Autodesk Inventor part; units mm, degrees
(part 2 of 11)
  arc A198 (21.2642, 29.6462) -> (21.4078, 29.7898) centre (21.336, 29.718) ccw
  line L98 (18.542, 32.512) -> (18.542, 37.846)
  arc A199 (18.6436, 37.846) -> (18.4404, 37.846) centre (18.542, 37.846) ccw
  arc A200 (18.4404, 32.512) -> (18.6436, 32.512) centre (18.542, 32.512) ccw
  line L99 (18.542, 37.846) -> (-1.016, 37.846)
  arc A201 (-1.016, 37.9476) -> (-1.016, 37.7444) centre (-1.016, 37.846) ccw
  arc A202 (18.542, 37.7444) -> (18.542, 37.9476) centre (18.542, 37.846) ccw
  line L100 (-1.016, 37.846) -> (-1.016, -0.762)
  arc A203 (-1.1176, -0.762) -> (-0.9144, -0.762) centre (-1.016, -0.762) ccw
  arc A204 (-0.9144, 37.846) -> (-1.1176, 37.846) centre (-1.016, 37.846) ccw
  line L101 (26.162, 10.668) -> (27.432, 10.668)
  arc A205 (27.432, 10.6045) -> (27.432, 10.7315) centre (27.432, 10.668) ccw
  arc A206 (26.162, 10.7315) -> (26.162, 10.6045) centre (26.162, 10.668) ccw
  line L102 (26.162, 26.162) -> (26.162, 27.432)
  arc A207 (26.2255, 27.432) -> (26.0985, 27.432) centre (26.162, 27.432) ccw
  arc A208 (26.0985, 26.162) -> (26.2255, 26.162) centre (26.162, 26.162) ccw
  line L103 (10.668, 26.162) -> (9.398, 26.162)
  arc A209 (9.398, 26.2255) -> (9.398, 26.0985) centre (9.398, 26.162) ccw
  arc A210 (10.668, 26.0985) -> (10.668, 26.2255) centre (10.668, 26.162) ccw
  line L104 (10.668, 10.668) -> (10.668, 9.398)
  arc A211 (10.6045, 9.398) -> (10.7315, 9.398) centre (10.668, 9.398) ccw
  arc A212 (10.7315, 10.668) -> (10.6045, 10.668) centre (10.668, 10.668) ccw
  line L105 (10.668, 26.162) -> (10.922, 26.162)
  arc A213 (10.922, 26.0985) -> (10.922, 26.2255) centre (10.922, 26.162) ccw
  arc A214 (10.668, 26.2255) -> (10.668, 26.0985) centre (10.668, 26.162) ccw
  line L106 (12.954, 26.67) -> (11.176, 26.67)
  arc A215 (11.176, 26.7335) -> (11.176, 26.6065) centre (11.176, 26.67) ccw
  arc A216 (12.954, 26.6065) -> (12.954, 26.7335) centre (12.954, 26.67) ccw
  line L107 (11.176, 26.67) -> (10.668, 26.162)
  arc A217 (10.6231, 26.2069) -> (10.7129, 26.1171) centre (10.668, 26.162) ccw
  arc A218 (11.2209, 26.6251) -> (11.1311, 26.7149) centre (11.176, 26.67) ccw
  line L108 (5.588, 34.036) -> (5.588, 30.48)
  arc A219 (5.5245, 30.48) -> (5.6515, 30.48) centre (5.588, 30.48) ccw
  arc A220 (5.6515, 34.036) -> (5.5245, 34.036) centre (5.588, 34.036) ccw
  line L109 (5.588, 30.48) -> (4.572, 29.464)
  arc A221 (4.5271, 29.5089) -> (4.6169, 29.4191) centre (4.572, 29.464) ccw
  arc A222 (5.6329, 30.4351) -> (5.5431, 30.5249) centre (5.588, 30.48) ccw
  line L110 (4.572, 29.464) -> (4.572, 23.368)
  arc A223 (4.5085, 23.368) -> (4.6355, 23.368) centre (4.572, 23.368) ccw
  arc A224 (4.6355, 29.464) -> (4.5085, 29.464) centre (4.572, 29.464) ccw
  line L111 (4.572, 23.368) -> (8.382, 19.558)
  arc A225 (8.3371, 19.5131) -> (8.4269, 19.6029) centre (8.382, 19.558) ccw
  arc A226 (4.6169, 23.4129) -> (4.5271, 23.3231) centre (4.572, 23.368) ccw
  line L112 (8.382, 19.558) -> (14.224, 19.558)
  arc A227 (14.224, 19.4945) -> (14.224, 19.6215) centre (14.224, 19.558) ccw
  arc A228 (8.382, 19.6215) -> (8.382, 19.4945) centre (8.382, 19.558) ccw
  line L113 (14.224, 19.558) -> (17.018, 22.352)
  arc A229 (17.0629, 22.3071) -> (16.9731, 22.3969) centre (17.018, 22.352) ccw
  arc A230 (14.1791, 19.6029) -> (14.2689, 19.5131) centre (14.224, 19.558) ccw
  line L114 (11.176, 20.32) -> (13.208, 20.32)
  arc A231 (13.208, 20.2565) -> (13.208, 20.3835) centre (13.208, 20.32) ccw
  arc A232 (11.176, 20.3835) -> (11.176, 20.2565) centre (11.176, 20.32) ccw
  line L115 (13.208, 20.32) -> (14.986, 22.098)
  arc A233 (15.0309, 22.0531) -> (14.9411, 22.1429) centre (14.986, 22.098) ccw
  arc A234 (13.1631, 20.3649) -> (13.2529, 20.2751) centre (13.208, 20.32) ccw
  line L116 (30.988, 34.29) -> (25.654, 34.29)
  arc A235 (25.654, 34.3535) -> (25.654, 34.2265) centre (25.654, 34.29) ccw
  arc A236 (30.988, 34.2265) -> (30.988, 34.3535) centre (30.988, 34.29) ccw
  line L117 (25.654, 34.29) -> (21.082, 29.718)
  arc A237 (21.0371, 29.7629) -> (21.1269, 29.6731) centre (21.082, 29.718) ccw
  arc A238 (25.6989, 34.2451) -> (25.6091, 34.3349) centre (25.654, 34.29) ccw
  line L118 (21.082, 29.718) -> (16.002, 29.718)
  arc A239 (16.002, 29.7815) -> (16.002, 29.6545) centre (16.002, 29.718) ccw
  arc A240 (21.082, 29.6545) -> (21.082, 29.7815) centre (21.082, 29.718) ccw
  line L119 (16.002, 29.718) -> (15.494, 30.226)
  arc A241 (15.5389, 30.2709) -> (15.4491, 30.1811) centre (15.494, 30.226) ccw
  arc A242 (15.9571, 29.6731) -> (16.0469, 29.7629) centre (16.002, 29.718) ccw
  line L120 (26.0801, 28.3448) -> (26.177, 28.9906)
  arc A243 (26.2147, 28.9849) -> (26.1802, 29.0285) centre (26.177, 28.9906) ccw
  arc A244 (26.0833, 28.3828) -> (26.0769, 28.3069) centre (26.0801, 28.3448) ccw
  line L121 (26.177, 28.9906) -> (26.3574, 29.6181)
  arc A245 (26.394, 29.6076) -> (26.3655, 29.6553) centre (26.3574, 29.6181) ccw
  arc A246 (26.1404, 29.0011) -> (26.1689, 28.9533) centre (26.177, 28.9906) ccw
  line L122 (26.3574, 29.6181) -> (26.6182, 30.2168)
  arc A247 (26.6053, 30.1809) -> (26.6311, 30.2526) centre (26.6182, 30.2168) ccw
  arc A248 (26.3225, 29.6333) -> (26.3445, 29.5823) centre (26.3574, 29.6181) ccw
  line L123 (26.6182, 30.2168) -> (26.9548, 30.7763)
  arc A249 (26.9374, 30.7424) -> (26.9723, 30.8101) centre (26.9548, 30.7763) ccw
  arc A250 (26.6356, 30.2506) -> (26.6007, 30.1829) centre (26.6182, 30.2168) ccw
  line L124 (26.9548, 30.7763) -> (29.3598, 30.1565)
  arc A251 (29.3381, 30.1252) -> (29.3815, 30.1878) centre (29.3598, 30.1565) ccw
  arc A252 (26.9766, 30.8075) -> (26.9331, 30.745) centre (26.9548, 30.7763) ccw
  line L125 (29.3598, 30.1565) -> (29.843, 29.7173)
  arc A253 (29.8174, 29.6891) -> (29.8686, 29.7455) centre (29.843, 29.7173) ccw
  arc A254 (29.3854, 30.1847) -> (29.3342, 30.1283) centre (29.3598, 30.1565) ccw
  line L126 (29.843, 29.7173) -> (30.2647, 29.2188)
  arc A255 (30.2356, 29.1942) -> (30.2938, 29.2434) centre (30.2647, 29.2188) ccw
  arc A256 (29.8721, 29.7419) -> (29.8139, 29.6927) centre (29.843, 29.7173) ccw
  line L127 (30.2647, 29.2188) -> (30.6178, 28.6694)
  arc A257 (30.5857, 28.6489) -> (30.6498, 28.6901) centre (30.6178, 28.6694) ccw
  arc A258 (30.2968, 29.2394) -> (30.2327, 29.1982) centre (30.2647, 29.2188) ccw
  line L128 (30.6178, 28.6694) -> (30.8961, 28.0788)
  arc A259 (30.8616, 28.0625) -> (30.9306, 28.095) centre (30.8961, 28.0788) ccw
  arc A260 (30.6522, 28.6857) -> (30.5833, 28.6532) centre (30.6178, 28.6694) ccw
  line L129 (30.8961, 28.0788) -> (31.0949, 27.4568)
  arc A261 (31.0586, 27.4452) -> (31.1312, 27.4684) centre (31.0949, 27.4568) ccw
  arc A262 (30.9324, 28.0903) -> (30.8598, 28.0672) centre (30.8961, 28.0788) ccw
  line L130 (31.0949, 27.4568) -> (31.2111, 26.8142)
  arc A263 (31.1736, 26.8075) -> (31.2486, 26.821) centre (31.2111, 26.8142) ccw
  arc A264 (31.1324, 27.4636) -> (31.0574, 27.45) centre (31.0949, 27.4568) ccw
  line L131 (31.2111, 26.8142) -> (31.2392, 26.1619)
  arc A265 (31.2012, 26.1601) -> (31.2773, 26.1637) centre (31.2392, 26.1619) ccw
  arc A266 (31.2491, 26.8161) -> (31.173, 26.8124) centre (31.2111, 26.8142) ccw
  line L132 (31.2392, 26.1619) -> (31.2053, 25.5496)
  arc A267 (31.1673, 25.5519) -> (31.2433, 25.5473) centre (31.2053, 25.5496) ccw
  arc A268 (31.2773, 26.1596) -> (31.2012, 26.1642) centre (31.2392, 26.1619) ccw
  line L133 (31.2053, 25.5496) -> (31.0945, 24.9462)
  arc A269 (31.0569, 24.9531) -> (31.1319, 24.9394) centre (31.0944, 24.9463) ccw
  arc A270 (31.2428, 25.5427) -> (31.1678, 25.5565) centre (31.2053, 25.5496) ccw
  line L134 (31.0945, 24.9462) -> (30.9118, 24.3606)
  arc A271 (30.8754, 24.372) -> (30.9482, 24.3493) centre (30.9118, 24.3606) ccw
  arc A272 (31.1309, 24.9349) -> (31.0581, 24.9576) centre (31.0945, 24.9462) ccw
  line L135 (30.9118, 24.3606) -> (30.6601, 23.8012)
  arc A273 (30.6253, 23.8168) -> (30.6948, 23.7856) centre (30.6601, 23.8012) ccw
  arc A274 (30.9465, 24.345) -> (30.877, 24.3763) centre (30.9118, 24.3606) ccw
  line L136 (30.6601, 23.8012) -> (30.3428, 23.2762)
  arc A275 (30.3102, 23.2959) -> (30.3754, 23.2565) centre (30.3428, 23.2762) ccw
  arc A276 (30.6927, 23.7815) -> (30.6275, 23.8209) centre (30.6601, 23.8012) ccw
  line L137 (30.3428, 23.2762) -> (29.9645, 22.7933)
  arc A277 (29.9345, 22.8168) -> (29.9945, 22.7698) centre (29.9645, 22.7933) ccw
  arc A278 (30.3728, 23.2527) -> (30.3128, 23.2997) centre (30.3428, 23.2762) ccw
  line L138 (29.9645, 22.7933) -> (29.5307, 22.3596)
  arc A279 (29.5037, 22.3865) -> (29.5576, 22.3326) centre (29.5307, 22.3596) ccw
  arc A280 (29.9914, 22.7664) -> (29.9375, 22.8203) centre (29.9645, 22.7933) ccw
  line L139 (29.5307, 22.3596) -> (29.0478, 21.9812)
  arc A281 (29.0243, 22.0112) -> (29.0713, 21.9512) centre (29.0478, 21.9812) ccw
  arc A282 (29.5542, 22.3296) -> (29.5072, 22.3896) centre (29.5307, 22.3596) ccw
  line L140 (29.0478, 21.9812) -> (28.5228, 21.6639)
  arc A283 (28.5031, 21.6965) -> (28.5425, 21.6313) centre (28.5228, 21.6639) ccw
  arc A284 (29.0675, 21.9486) -> (29.0281, 22.0138) centre (29.0478, 21.9812) ccw
  line L141 (28.5228, 21.6639) -> (27.9634, 21.4121)
  arc A285 (27.9478, 21.4469) -> (27.9791, 21.3774) centre (27.9634, 21.4121) ccw
  arc A286 (28.5384, 21.6291) -> (28.5072, 21.6986) centre (28.5228, 21.6639) ccw
  line L142 (27.9634, 21.4121) -> (27.3777, 21.2296)
  arc A287 (27.3664, 21.266) -> (27.3891, 21.1933) centre (27.3777, 21.2296) ccw
  arc A288 (27.9747, 21.3758) -> (27.9521, 21.4485) centre (27.9634, 21.4121) ccw
  line L143 (27.3777, 21.2296) -> (26.7743, 21.119)
  arc A289 (26.7675, 21.1565) -> (26.7812, 21.0816) centre (26.7743, 21.119) ccw
  arc A290 (27.3846, 21.1921) -> (27.3709, 21.2671) centre (27.3777, 21.2296) ccw
  line L144 (26.7743, 21.119) -> (26.162, 21.082)
  arc A291 (26.1597, 21.12) -> (26.1643, 21.044) centre (26.162, 21.082) ccw
  arc A292 (26.7766, 21.081) -> (26.772, 21.1571) centre (26.7743, 21.119) ccw
  line L145 (26.162, 21.082) -> (25.5497, 21.119)
  arc A293 (25.552, 21.1571) -> (25.5474, 21.081) centre (25.5497, 21.119) ccw
  arc A294 (26.1597, 21.044) -> (26.1643, 21.12) centre (26.162, 21.082) ccw
  line L146 (25.5497, 21.119) -> (24.9463, 21.2296)
  arc A295 (24.9531, 21.2671) -> (24.9394, 21.1921) centre (24.9463, 21.2296) ccw
  arc A296 (25.5428, 21.0816) -> (25.5565, 21.1565) centre (25.5497, 21.119) ccw
  line L147 (24.9463, 21.2296) -> (24.3606, 21.4121)
  arc A297 (24.3719, 21.4485) -> (24.3493, 21.3758) centre (24.3606, 21.4121) ccw
  arc A298 (24.935, 21.1933) -> (24.9576, 21.266) centre (24.9463, 21.2296) ccw
  line L148 (24.3606, 21.4121) -> (23.8012, 21.6639)
  arc A299 (23.8168, 21.6986) -> (23.7856, 21.6291) centre (23.8012, 21.6639) ccw
  arc A300 (24.345, 21.3774) -> (24.3763, 21.4469) centre (24.3606, 21.4121) ccw
  line L149 (23.8012, 21.6639) -> (23.2762, 21.9812)
  arc A301 (23.2959, 22.0138) -> (23.2565, 21.9486) centre (23.2762, 21.9812) ccw
  arc A302 (23.7815, 21.6313) -> (23.8209, 21.6965) centre (23.8012, 21.6639) ccw
  line L150 (23.2762, 21.9812) -> (22.7933, 22.3596)
  arc A303 (22.8168, 22.3896) -> (22.7698, 22.3296) centre (22.7933, 22.3596) ccw
  arc A304 (23.2527, 21.9512) -> (23.2997, 22.0112) centre (23.2762, 21.9812) ccw
  line L151 (22.7933, 22.3596) -> (22.3596, 22.7933)
  arc A305 (22.3865, 22.8203) -> (22.3326, 22.7664) centre (22.3596, 22.7933) ccw
  arc A306 (22.7664, 22.3326) -> (22.8203, 22.3865) centre (22.7933, 22.3596) ccw
  line L152 (22.3596, 22.7933) -> (21.9812, 23.2762)
  arc A307 (22.0112, 23.2997) -> (21.9512, 23.2527) centre (21.9812, 23.2762) ccw
  arc A308 (22.3296, 22.7698) -> (22.3896, 22.8168) centre (22.3596, 22.7933) ccw
  line L153 (21.9812, 23.2762) -> (21.6639, 23.8012)
  arc A309 (21.6965, 23.8209) -> (21.6313, 23.7815) centre (21.6639, 23.8012) ccw
  arc A310 (21.9486, 23.2565) -> (22.0139, 23.2959) centre (21.9812, 23.2762) ccw
  line L154 (21.6639, 23.8012) -> (21.4121, 24.3606)
  arc A311 (21.4469, 24.3763) -> (21.3774, 24.345) centre (21.4121, 24.3606) ccw
  arc A312 (21.6291, 23.7856) -> (21.6986, 23.8168) centre (21.6639, 23.8012) ccw
  line L155 (21.4121, 24.3606) -> (21.2296, 24.9463)
  arc A313 (21.266, 24.9576) -> (21.1933, 24.935) centre (21.2296, 24.9463) ccw
  arc A314 (21.3758, 24.3493) -> (21.4485, 24.3719) centre (21.4121, 24.3606) ccw
  line L156 (21.2296, 24.9463) -> (21.119, 25.5497)
  arc A315 (21.1565, 25.5565) -> (21.0816, 25.5428) centre (21.119, 25.5497) ccw
  arc A316 (21.1921, 24.9394) -> (21.2671, 24.9531) centre (21.2296, 24.9463) ccw
  line L157 (21.119, 25.5497) -> (21.082, 26.162)
  arc A317 (21.12, 26.1643) -> (21.044, 26.1597) centre (21.082, 26.162) ccw
  arc A318 (21.081, 25.5474) -> (21.1571, 25.552) centre (21.119, 25.5497) ccw
  line L158 (21.082, 26.162) -> (21.1406, 26.8194)
  arc A319 (21.1786, 26.816) -> (21.1027, 26.8228) centre (21.1406, 26.8194) ccw
  arc A320 (21.0441, 26.1654) -> (21.1199, 26.1586) centre (21.082, 26.162) ccw
  line L159 (21.1406, 26.8194) -> (21.2818, 27.464)
  arc A321 (21.319, 27.4559) -> (21.2446, 27.4722) centre (21.2818, 27.464) ccw
  arc A322 (21.1034, 26.8275) -> (21.1778, 26.8112) centre (21.1406, 26.8194) ccw
  line L160 (21.2818, 27.464) -> (21.5033, 28.0857)
  arc A323 (21.5392, 28.073) -> (21.4674, 28.0985) centre (21.5033, 28.0857) ccw
  arc A324 (21.2459, 27.4768) -> (21.3177, 27.4513) centre (21.2818, 27.464) ccw
  line L161 (21.5033, 28.0857) -> (21.8015, 28.6745)
  arc A325 (21.8355, 28.6573) -> (21.7675, 28.6917) centre (21.8015, 28.6745) ccw
  arc A326 (21.4693, 28.103) -> (21.5373, 28.0685) centre (21.5033, 28.0857) ccw
  line L162 (21.8015, 28.6745) -> (22.1716, 29.2209)
  arc A327 (22.2032, 29.1995) -> (22.1401, 29.2422) centre (22.1716, 29.2209) ccw
  arc A328 (21.7699, 28.6959) -> (21.833, 28.6532) centre (21.8015, 28.6745) ccw
  line L163 (22.1716, 29.2209) -> (22.6078, 29.7162)
  arc A329 (22.6364, 29.691) -> (22.5793, 29.7413) centre (22.6078, 29.7162) ccw
  arc A330 (22.143, 29.2461) -> (22.2002, 29.1957) centre (22.1716, 29.2209) ccw
  line L164 (22.6078, 29.7162) -> (23.1031, 30.1524)
  arc A331 (23.1283, 30.1238) -> (23.0779, 30.181) centre (23.1031, 30.1524) ccw
  arc A332 (22.5827, 29.7447) -> (22.633, 29.6876) centre (22.6078, 29.7162) ccw
  line L165 (23.1031, 30.1524) -> (23.6495, 30.5225)
  arc A333 (23.6708, 30.491) -> (23.6281, 30.5541) centre (23.6495, 30.5225) ccw
  arc A334 (23.0817, 30.1839) -> (23.1245, 30.1208) centre (23.1031, 30.1524) ccw
  line L166 (23.6495, 30.5225) -> (24.2383, 30.8207)
  arc A335 (24.2555, 30.7867) -> (24.221, 30.8547) centre (24.2382, 30.8207) ccw
  arc A336 (23.6323, 30.5565) -> (23.6667, 30.4885) centre (23.6495, 30.5225) ccw
  line L167 (24.2383, 30.8207) -> (24.8599, 31.0422)
  arc A337 (24.8727, 31.0063) -> (24.8472, 31.0781) centre (24.8599, 31.0422) ccw
  arc A338 (24.2255, 30.8566) -> (24.251, 30.7848) centre (24.2382, 30.8207) ccw
  line L168 (24.8599, 31.0422) -> (25.5046, 31.1834)
  arc A339 (25.5128, 31.1462) -> (25.4965, 31.2206) centre (25.5046, 31.1834) ccw
  arc A340 (24.8518, 31.0794) -> (24.8681, 31.005) centre (24.8599, 31.0422) ccw
  line L169 (25.5046, 31.1834) -> (26.162, 31.242)
  arc A341 (26.1654, 31.2041) -> (26.1586, 31.28) centre (26.162, 31.242) ccw
  arc A342 (25.5012, 31.2213) -> (25.508, 31.1454) centre (25.5046, 31.1834) ccw
  line L170 (26.162, 31.242) -> (26.162, 29.972)
  arc A343 (26.1239, 29.972) -> (26.2001, 29.972) centre (26.162, 29.972) ccw
  arc A344 (26.2001, 31.242) -> (26.1239, 31.242) centre (26.162, 31.242) ccw
  line L171 (26.162, 29.972) -> (25.6365, 29.9526)
  arc A345 (25.6352, 29.9907) -> (25.638, 29.9145) centre (25.6366, 29.9526) ccw
  arc A346 (26.1634, 29.9339) -> (26.1606, 30.0101) centre (26.162, 29.972) ccw
  line L172 (25.6365, 29.9526) -> (25.1192, 29.8586)
  arc A347 (25.1124, 29.8961) -> (25.126, 29.8211) centre (25.1192, 29.8586) ccw
  arc A348 (25.6434, 29.9151) -> (25.6297, 29.9901) centre (25.6366, 29.9526) ccw
  line L173 (25.1192, 29.8586) -> (24.6206, 29.6919)
  arc A349 (24.6085, 29.7281) -> (24.6326, 29.6558) centre (24.6206, 29.6919) ccw
  arc A350 (25.1313, 29.8225) -> (25.1072, 29.8947) centre (25.1192, 29.8586) ccw
  line L174 (24.6206, 29.6919) -> (24.1507, 29.456)
  arc A351 (24.1336, 29.49) -> (24.1677, 29.4219) centre (24.1506, 29.456) ccw
  arc A352 (24.6376, 29.6579) -> (24.6035, 29.726) centre (24.6206, 29.6919) ccw
  line L175 (24.1507, 29.456) -> (23.7191, 29.1556)
  arc A353 (23.6974, 29.1868) -> (23.7409, 29.1243) centre (23.7191, 29.1556) ccw
  arc A354 (24.1724, 29.4247) -> (24.1289, 29.4873) centre (24.1507, 29.456) ccw
  line L176 (23.7191, 29.1556) -> (23.3348, 28.7968)
  arc A355 (23.3087, 28.8247) -> (23.3607, 28.769) centre (23.3347, 28.7968) ccw
  arc A356 (23.7451, 29.1277) -> (23.6931, 29.1834) centre (23.7191, 29.1556) ccw
  line L177 (23.3348, 28.7968) -> (23.0053, 28.387)
  arc A357 (22.9756, 28.4109) -> (23.035, 28.3631) centre (23.0053, 28.387) ccw
  arc A358 (23.3644, 28.773) -> (23.305, 28.8207) centre (23.3347, 28.7968) ccw
  line L178 (23.0053, 28.387) -> (22.7376, 27.9345)
  arc A359 (22.7048, 27.9539) -> (22.7704, 27.9151) centre (22.7376, 27.9345) ccw
  arc A360 (23.0381, 28.3676) -> (22.9725, 28.4064) centre (23.0053, 28.387) ccw
  line L179 (22.7376, 27.9345) -> (22.5369, 27.4485)
  arc A361 (22.5018, 27.463) -> (22.5722, 27.4339) centre (22.537, 27.4485) ccw
  arc A362 (22.7728, 27.92) -> (22.7024, 27.949) centre (22.7376, 27.9345) ccw
  line L180 (22.5369, 27.4485) -> (22.4076, 26.9389)
  arc A363 (22.3706, 26.9482) -> (22.4445, 26.9295) centre (22.4076, 26.9388) ccw
  arc A364 (22.5739, 27.4391) -> (22.5, 27.4579) centre (22.5369, 27.4485) ccw
  line L181 (22.4076, 26.9389) -> (22.352, 26.416)
  arc A365 (22.3141, 26.42) -> (22.3899, 26.412) centre (22.352, 26.416) ccw
  arc A366 (22.4454, 26.9348) -> (22.3697, 26.9429) centre (22.4076, 26.9388) ccw
  line L182 (22.352, 26.416) -> (22.352, 26.162)
  arc A367 (22.3139, 26.162) -> (22.3901, 26.162) centre (22.352, 26.162) ccw
  arc A368 (22.3901, 26.416) -> (22.3139, 26.416) centre (22.352, 26.416) ccw
  line L183 (22.352, 26.162) -> (22.3908, 25.6198)
  arc A369 (22.3528, 25.6171) -> (22.4288, 25.6225) centre (22.3908, 25.6198) ccw
  arc A370 (22.39, 26.1647) -> (22.314, 26.1593) centre (22.352, 26.162) ccw
  line L184 (22.3908, 25.6198) -> (22.5063, 25.0886)
  arc A371 (22.4691, 25.0805) -> (22.5436, 25.0967) centre (22.5063, 25.0886) ccw
  arc A372 (22.428, 25.6279) -> (22.3536, 25.6117) centre (22.3908, 25.6198) ccw
  line L185 (22.5063, 25.0886) -> (22.6963, 24.5793)
  arc A373 (22.6606, 24.566) -> (22.732, 24.5926) centre (22.6963, 24.5793) ccw
  arc A374 (22.542, 25.1019) -> (22.4706, 25.0753) centre (22.5063, 25.0886) ccw
  line L186 (22.6963, 24.5793) -> (22.9568, 24.1022)
  arc A375 (22.9234, 24.0839) -> (22.9903, 24.1204) centre (22.9568, 24.1022) ccw
  arc A376 (22.7297, 24.5975) -> (22.6629, 24.561) centre (22.6963, 24.5793) ccw
  line L187 (22.9568, 24.1022) -> (23.2827, 23.6671)
  arc A377 (23.2521, 23.6441) -> (23.3131, 23.6898) centre (23.2826, 23.667) ccw
  arc A378 (22.9873, 24.125) -> (22.9263, 24.0793) centre (22.9568, 24.1022) ccw
  line L188 (23.2827, 23.6671) -> (23.667, 23.2826)
  arc A379 (23.64, 23.2557) -> (23.6939, 23.3095) centre (23.667, 23.2826) ccw
  arc A380 (23.3095, 23.6939) -> (23.2557, 23.64) centre (23.2826, 23.667) ccw
  line L189 (23.667, 23.2826) -> (24.1022, 22.9568)
  arc A381 (24.0793, 22.9263) -> (24.125, 22.9873) centre (24.1022, 22.9568) ccw
  arc A382 (23.6898, 23.3131) -> (23.6441, 23.2521) centre (23.667, 23.2826) ccw
  line L190 (24.1022, 22.9568) -> (24.5793, 22.6963)
  arc A383 (24.561, 22.6629) -> (24.5975, 22.7297) centre (24.5793, 22.6963) ccw
  arc A384 (24.1204, 22.9903) -> (24.0839, 22.9234) centre (24.1022, 22.9568) ccw
  line L191 (24.5793, 22.6963) -> (25.0886, 22.5063)
  arc A385 (25.0753, 22.4706) -> (25.1019, 22.542) centre (25.0886, 22.5063) ccw
  arc A386 (24.5926, 22.732) -> (24.566, 22.6606) centre (24.5793, 22.6963) ccw
  line L192 (25.0886, 22.5063) -> (25.6198, 22.3908)
  arc A387 (25.6117, 22.3536) -> (25.6279, 22.428) centre (25.6198, 22.3908) ccw
  arc A388 (25.0967, 22.5436) -> (25.0805, 22.4691) centre (25.0886, 22.5063) ccw
  line L193 (25.6198, 22.3908) -> (26.162, 22.352)
  arc A389 (26.1593, 22.314) -> (26.1647, 22.39) centre (26.162, 22.352) ccw
  line L194 (23.0121, 24.0284) -> (21.5616, 24.0284)
  line L195 (26.162, 22.352) -> (26.7042, 22.3908)
  arc A390 (26.7069, 22.3528) -> (26.7015, 22.4288) centre (26.7042, 22.3908) ccw
  arc A391 (26.1593, 22.39) -> (26.1647, 22.314) centre (26.162, 22.352) ccw
  line L196 (26.7042, 22.3908) -> (27.2354, 22.5063)
  arc A392 (27.2435, 22.4691) -> (27.2273, 22.5436) centre (27.2354, 22.5063) ccw
  arc A393 (26.6961, 22.428) -> (26.7123, 22.3535) centre (26.7042, 22.3908) ccw
  line L197 (27.2354, 22.5063) -> (27.7447, 22.6963)
  arc A394 (27.758, 22.6606) -> (27.7314, 22.732) centre (27.7447, 22.6963) ccw
  arc A395 (27.2221, 22.542) -> (27.2487, 22.4706) centre (27.2354, 22.5063) ccw
  line L198 (27.7447, 22.6963) -> (28.2218, 22.9568)
  arc A396 (28.2401, 22.9234) -> (28.2036, 22.9903) centre (28.2218, 22.9568) ccw
  arc A397 (27.7265, 22.7297) -> (27.763, 22.6629) centre (27.7447, 22.6963) ccw
  line L199 (28.2218, 22.9568) -> (28.657, 23.2826)
  arc A398 (28.6799, 23.2521) -> (28.6342, 23.3131) centre (28.657, 23.2826) ccw
  arc A399 (28.199, 22.9873) -> (28.2447, 22.9263) centre (28.2218, 22.9568) ccw
  line L200 (28.657, 23.2826) -> (29.0414, 23.667)
  arc A400 (29.0683, 23.64) -> (29.0145, 23.6939) centre (29.0414, 23.667) ccw
  arc A401 (28.6301, 23.3095) -> (28.684, 23.2557) centre (28.657, 23.2826) ccw
  line L201 (29.0414, 23.667) -> (29.3672, 24.1022)
  arc A402 (29.3977, 24.0793) -> (29.3367, 24.125) centre (29.3672, 24.1022) ccw
  arc A403 (29.0109, 23.6898) -> (29.0719, 23.6441) centre (29.0414, 23.667) ccw
  line L202 (29.3672, 24.1022) -> (29.6277, 24.5793)
  arc A404 (29.6611, 24.561) -> (29.5943, 24.5975) centre (29.6277, 24.5793) ccw
  arc A405 (29.3337, 24.1204) -> (29.4006, 24.0839) centre (29.3672, 24.1022) ccw
  line L203 (29.6277, 24.5793) -> (29.8177, 25.0886)
  arc A406 (29.8534, 25.0753) -> (29.782, 25.1019) centre (29.8177, 25.0886) ccw
  arc A407 (29.592, 24.5926) -> (29.6634, 24.566) centre (29.6277, 24.5793) ccw
  line L204 (29.8177, 25.0886) -> (29.9332, 25.6198)
  arc A408 (29.9704, 25.6117) -> (29.896, 25.6279) centre (29.9332, 25.6198) ccw
  arc A409 (29.7804, 25.0967) -> (29.8549, 25.0805) centre (29.8177, 25.0886) ccw
  line L205 (29.9332, 25.6198) -> (29.972, 26.162)
  arc A410 (30.01, 26.1593) -> (29.934, 26.1647) centre (29.972, 26.162) ccw
  arc A411 (29.8952, 25.6225) -> (29.9712, 25.6171) centre (29.9332, 25.6198) ccw
  line L206 (29.972, 26.162) -> (29.9518, 26.6485)
  arc A412 (29.9898, 26.65) -> (29.9137, 26.6469) centre (29.9518, 26.6485) ccw
  arc A413 (29.9339, 26.1604) -> (30.0101, 26.1636) centre (29.972, 26.162) ccw
  line L207 (29.9518, 26.6485) -> (29.8682, 27.1281)
  arc A414 (29.9058, 27.1347) -> (29.8307, 27.1216) centre (29.8682, 27.1281) ccw
  arc A415 (29.9142, 26.6419) -> (29.9893, 26.655) centre (29.9518, 26.6485) ccw
  line L208 (29.8682, 27.1281) -> (29.7228, 27.5928)
  arc A416 (29.7591, 27.6042) -> (29.6864, 27.5814) centre (29.7228, 27.5928) ccw
  arc A417 (29.8318, 27.1167) -> (29.9046, 27.1395) centre (29.8682, 27.1281) ccw
  line L209 (29.7228, 27.5928) -> (29.5179, 28.0345)
  arc A418 (29.5525, 28.0505) -> (29.4834, 28.0184) centre (29.5179, 28.0345) ccw
  arc A419 (29.6882, 27.5767) -> (29.7574, 27.6088) centre (29.7228, 27.5928) ccw
  line L210 (29.5179, 28.0345) -> (29.2572, 28.4456)
  arc A420 (29.2893, 28.466) -> (29.225, 28.4252) centre (29.2572, 28.4456) ccw
  arc A421 (29.4857, 28.0141) -> (29.5501, 28.0549) centre (29.5179, 28.0345) ccw
  line L211 (29.2572, 28.4456) -> (28.945, 28.8193)
  arc A422 (28.9742, 28.8437) -> (28.9157, 28.7948) centre (28.945, 28.8193) ccw
  arc A423 (29.2279, 28.4212) -> (29.2864, 28.4701) centre (29.2572, 28.4456) ccw
  line L212 (28.945, 28.8193) -> (28.5867, 29.1489)
  arc A424 (28.6125, 29.177) -> (28.5609, 29.1209) centre (28.5867, 29.1489) ccw
  arc A425 (28.9192, 28.7912) -> (28.9708, 28.8473) centre (28.945, 28.8193) ccw
  line L213 (28.5867, 29.1489) -> (28.1884, 29.429)
  arc A426 (28.2104, 29.4602) -> (28.1665, 29.3979) centre (28.1884, 29.429) ccw
  arc A427 (28.5648, 29.1178) -> (28.6086, 29.1801) centre (28.5867, 29.1489) ccw
  line L214 (28.1884, 29.429) -> (27.757, 29.6547)
  arc A428 (27.7747, 29.6885) -> (27.7394, 29.621) centre (27.757, 29.6547) ccw
  arc A429 (28.1708, 29.3953) -> (28.2061, 29.4628) centre (28.1884, 29.429) ccw
  line L215 (27.757, 29.6547) -> (27.5599, 29.2096)
  arc A430 (27.313, 29.858) -> (27.2868, 29.7864) centre (27.2999, 29.8222) ccw
  arc A431 (27.7439, 29.619) -> (27.7702, 29.6905) centre (27.757, 29.6547) ccw
  line L216 (27.5599, 29.2096) -> (27.4225, 28.7424)
  arc A432 (27.4309, 28.7796) -> (27.4142, 28.7052) centre (27.4225, 28.7424) ccw
  arc A433 (27.5516, 29.1724) -> (27.5682, 29.2467) centre (27.5599, 29.2095) ccw
  line L217 (27.4225, 28.7424) -> (27.3473, 28.2614)
  arc A434 (27.3507, 28.2993) -> (27.3439, 28.2235) centre (27.3473, 28.2614) ccw
  arc A435 (27.4191, 28.7045) -> (27.4259, 28.7804) centre (27.4225, 28.7424) ccw
  line L218 (27.3473, 28.2614) -> (26.0801, 28.3448)
  arc A436 (26.1182, 28.3448) -> (26.042, 28.3448) centre (26.0801, 28.3448) ccw
  arc A437 (27.3092, 28.2614) -> (27.3775, 28.2847) centre (27.3473, 28.2614) ccw
  line L219 (26.8494, 21.1328) -> (25.4746, 21.1328)
  arc A438 (25.4746, 21.1709) -> (25.4746, 21.0947) centre (25.4746, 21.1328) ccw
  arc A439 (26.8494, 21.0947) -> (26.8494, 21.1709) centre (26.8494, 21.1328) ccw
  line L220 (27.5561, 21.2852) -> (24.7679, 21.2852)
  arc A440 (24.7679, 21.3233) -> (24.7679, 21.2471) centre (24.7679, 21.2852) ccw
  arc A441 (27.5561, 21.2471) -> (27.5561, 21.3233) centre (27.5561, 21.2852) ccw
  line L221 (28.02, 21.4376) -> (24.304, 21.4376)
  arc A442 (24.304, 21.4757) -> (24.304, 21.3995) centre (24.304, 21.4376) ccw
  arc A443 (28.02, 21.3995) -> (28.02, 21.4757) centre (28.02, 21.4376) ccw
  line L222 (28.3587, 21.59) -> (23.9654, 21.59)
  arc A444 (23.9654, 21.6281) -> (23.9654, 21.5519) centre (23.9654, 21.59) ccw
  arc A445 (28.3587, 21.5519) -> (28.3587, 21.6281) centre (28.3587, 21.59) ccw
  line L223 (28.6527, 21.7424) -> (23.6713, 21.7424)
  arc A446 (23.6713, 21.7805) -> (23.6713, 21.7043) centre (23.6713, 21.7424) ccw
  arc A447 (28.6527, 21.7043) -> (28.6527, 21.7805) centre (28.6527, 21.7424) ccw
  line L224 (28.9048, 21.8948) -> (23.4192, 21.8948)
  arc A448 (23.4192, 21.9329) -> (23.4192, 21.8567) centre (23.4192, 21.8948) ccw
  arc A449 (28.9048, 21.8567) -> (28.9048, 21.9329) centre (28.9048, 21.8948) ccw
  line L225 (29.132, 22.0472) -> (23.1921, 22.0471)
  arc A450 (23.1921, 22.0852) -> (23.1921, 22.009) centre (23.1921, 22.0471) ccw
  arc A451 (29.132, 22.0091) -> (29.132, 22.0853) centre (29.132, 22.0472) ccw
  line L226 (29.3265, 22.1996) -> (22.9975, 22.1996)
  arc A452 (22.9975, 22.2377) -> (22.9975, 22.1615) centre (22.9975, 22.1996) ccw
  arc A453 (29.3265, 22.1615) -> (29.3265, 22.2377) centre (29.3265, 22.1996) ccw
  line L227 (29.521, 22.352) -> (26.162, 22.352)
  arc A454 (26.162, 22.3901) -> (26.162, 22.3139) centre (26.162, 22.352) ccw
  arc A455 (29.521, 22.3139) -> (29.521, 22.3901) centre (29.521, 22.352) ccw
  line L228 (26.162, 22.352) -> (22.803, 22.352)
  arc A456 (22.803, 22.3901) -> (22.803, 22.3139) centre (22.803, 22.352) ccw
  arc A457 (26.162, 22.3139) -> (26.162, 22.3901) centre (26.162, 22.352) ccw
  line L229 (29.6755, 22.5044) -> (27.2265, 22.5044)
  arc A458 (27.2265, 22.5425) -> (27.2265, 22.4663) centre (27.2265, 22.5044) ccw
  arc A459 (29.6755, 22.4663) -> (29.6755, 22.5425) centre (29.6755, 22.5044) ccw
  line L230 (25.0975, 22.5044) -> (22.6485, 22.5044)
  arc A460 (22.6485, 22.5425) -> (22.6485, 22.4663) centre (22.6485, 22.5044) ccw
  arc A461 (25.0975, 22.4663) -> (25.0975, 22.5425) centre (25.0975, 22.5044) ccw
  line L231 (29.8279, 22.6568) -> (27.6388, 22.6568)
  arc A462 (27.6388, 22.6949) -> (27.6388, 22.6187) centre (27.6388, 22.6568) ccw
  arc A463 (29.8279, 22.6187) -> (29.8279, 22.6949) centre (29.8279, 22.6568) ccw
  line L232 (24.6852, 22.6568) -> (22.4961, 22.6568)
  arc A464 (22.4961, 22.6949) -> (22.4961, 22.6187) centre (22.4961, 22.6568) ccw
  arc A465 (24.6852, 22.6187) -> (24.6852, 22.6949) centre (24.6852, 22.6568) ccw
  line L233 (29.9769, 22.8092) -> (27.9515, 22.8092)
  arc A466 (27.9515, 22.8473) -> (27.9515, 22.7711) centre (27.9515, 22.8092) ccw
  arc A467 (29.9769, 22.7711) -> (29.9769, 22.8473) centre (29.9769, 22.8092) ccw
  line L234 (24.3725, 22.8092) -> (22.3471, 22.8092)
  arc A468 (22.3471, 22.8473) -> (22.3471, 22.7711) centre (22.3471, 22.8092) ccw
  arc A469 (24.3725, 22.7711) -> (24.3725, 22.8473) centre (24.3725, 22.8092) ccw
  line L235 (30.0963, 22.9616) -> (28.2282, 22.9616)
  arc A470 (28.2282, 22.9997) -> (28.2282, 22.9235) centre (28.2282, 22.9616) ccw
  arc A471 (30.0963, 22.9235) -> (30.0963, 22.9997) centre (30.0963, 22.9616) ccw
  line L236 (24.0958, 22.9616) -> (22.2277, 22.9616)
  arc A472 (22.2277, 22.9997) -> (22.2277, 22.9235) centre (22.2277, 22.9616) ccw
  arc A473 (24.0958, 22.9235) -> (24.0958, 22.9997) centre (24.0958, 22.9616) ccw
  line L237 (30.2157, 23.114) -> (28.4318, 23.114)
  arc A474 (28.4318, 23.1521) -> (28.4318, 23.0759) centre (28.4318, 23.114) ccw
  arc A475 (30.2157, 23.0759) -> (30.2157, 23.1521) centre (30.2157, 23.114) ccw
  line L238 (23.8922, 23.114) -> (22.1083, 23.114)
  arc A476 (22.1083, 23.1521) -> (22.1083, 23.0759) centre (22.1083, 23.114) ccw
  arc A477 (23.8922, 23.0759) -> (23.8922, 23.1521) centre (23.8922, 23.114) ccw
  line L239 (30.3351, 23.2664) -> (28.6354, 23.2664)
  arc A478 (28.6354, 23.3045) -> (28.6354, 23.2283) centre (28.6354, 23.2664) ccw
  arc A479 (30.3351, 23.2283) -> (30.3351, 23.3045) centre (30.3351, 23.2664) ccw
  line L240 (23.6886, 23.2664) -> (21.9889, 23.2664)
  arc A480 (21.9889, 23.3045) -> (21.9889, 23.2283) centre (21.9889, 23.2664) ccw
  arc A481 (23.6886, 23.2283) -> (23.6886, 23.3045) centre (23.6886, 23.2664) ccw
  line L241 (30.429, 23.4188) -> (28.7933, 23.4186)
  arc A482 (28.7933, 23.4567) -> (28.7933, 23.3805) centre (28.7933, 23.4186) ccw
  arc A483 (30.429, 23.3807) -> (30.429, 23.4569) centre (30.429, 23.4188) ccw
  line L242 (23.5308, 23.4188) -> (21.8951, 23.4188)
  arc A484 (21.8951, 23.4569) -> (21.8951, 23.3807) centre (21.8951, 23.4188) ccw
  arc A485 (23.5308, 23.3807) -> (23.5308, 23.4569) centre (23.5308, 23.4188) ccw
  line L243 (30.5211, 23.5712) -> (28.9456, 23.571)
  arc A486 (28.9456, 23.6091) -> (28.9456, 23.5329) centre (28.9456, 23.571) ccw
  arc A487 (30.5211, 23.5331) -> (30.5211, 23.6093) centre (30.5211, 23.5712) ccw
  line L244 (23.3784, 23.5712) -> (21.8029, 23.5712)
  arc A488 (21.8029, 23.6093) -> (21.8029, 23.5331) centre (21.8029, 23.5712) ccw
  arc A489 (23.3784, 23.5331) -> (23.3784, 23.6093) centre (23.3784, 23.5712) ccw
  line L245 (30.6132, 23.7236) -> (29.0838, 23.7236)
  arc A490 (29.0838, 23.7617) -> (29.0838, 23.6855) centre (29.0838, 23.7236) ccw
  arc A491 (30.6132, 23.6855) -> (30.6132, 23.7617) centre (30.6132, 23.7236) ccw
  line L246 (23.2403, 23.7237) -> (21.7108, 23.7236)
  arc A492 (21.7108, 23.7617) -> (21.7108, 23.6855) centre (21.7108, 23.7236) ccw
  arc A493 (23.2403, 23.6856) -> (23.2403, 23.7618) centre (23.2403, 23.7237) ccw
  line L247 (30.6937, 23.876) -> (29.1979, 23.8758)
  arc A494 (29.1979, 23.9139) -> (29.1979, 23.8377) centre (29.1979, 23.8758) ccw
  arc A495 (30.6937, 23.8379) -> (30.6937, 23.9141) centre (30.6937, 23.876) ccw
  line L248 (23.1261, 23.876) -> (21.6302, 23.876)
  arc A496 (21.6302, 23.9141) -> (21.6302, 23.8379) centre (21.6302, 23.876) ccw
  arc A497 (23.1261, 23.8379) -> (23.1261, 23.9141) centre (23.1261, 23.876) ccw
  line L249 (30.7623, 24.0284) -> (29.312, 24.0284)
  arc A498 (29.312, 24.0665) -> (29.312, 23.9903) centre (29.312, 24.0284) ccw
  arc A499 (30.7623, 23.9903) -> (30.7623, 24.0665) centre (30.7623, 24.0284) ccw
  line L250 (23.0121, 24.0284) -> (21.5616, 24.0284)
  arc A500 (21.5616, 24.0665) -> (21.5616, 23.9903) centre (21.5616, 24.0284) ccw
  arc A501 (23.0121, 23.9903) -> (23.0121, 24.0665) centre (23.0121, 24.0284) ccw
  line L251 (30.8309, 24.1808) -> (29.4101, 24.1808)
  arc A502 (29.4101, 24.2189) -> (29.4101, 24.1427) centre (29.4101, 24.1808) ccw
  arc A503 (30.8309, 24.1427) -> (30.8309, 24.2189) centre (30.8309, 24.1808) ccw
  line L252 (22.9139, 24.1808) -> (21.4931, 24.1808)
  arc A504 (21.4931, 24.2189) -> (21.4931, 24.1427) centre (21.4931, 24.1808) ccw
  arc A505 (22.9139, 24.1427) -> (22.9139, 24.2189) centre (22.9139, 24.1808) ccw
  line L253 (30.8996, 24.3332) -> (29.4933, 24.3332)
  arc A506 (29.4933, 24.3713) -> (29.4933, 24.2951) centre (29.4933, 24.3332) ccw
  arc A507 (30.8996, 24.2951) -> (30.8996, 24.3713) centre (30.8996, 24.3332) ccw
  line L254 (22.8307, 24.3332) -> (21.4245, 24.3332)
  arc A508 (21.4245, 24.3713) -> (21.4245, 24.2951) centre (21.4245, 24.3332) ccw
  arc A509 (22.8307, 24.2951) -> (22.8307, 24.3713) centre (22.8307, 24.3332) ccw
  line L255 (30.9508, 24.4856) -> (29.5765, 24.4856)
  arc A510 (29.5765, 24.5237) -> (29.5765, 24.4475) centre (29.5765, 24.4856) ccw
  arc A511 (30.9508, 24.4475) -> (30.9508, 24.5237) centre (30.9508, 24.4856) ccw
  line L256 (22.7474, 24.4856) -> (21.3732, 24.4857)
  arc A512 (21.3732, 24.5238) -> (21.3732, 24.4476) centre (21.3732, 24.4857) ccw
  arc A513 (22.7474, 24.4475) -> (22.7474, 24.5237) centre (22.7474, 24.4856) ccw
  line L257 (30.9983, 24.638) -> (29.6496, 24.638)
  arc A514 (29.6496, 24.6761) -> (29.6496, 24.5999) centre (29.6496, 24.638) ccw
  arc A515 (30.9983, 24.5999) -> (30.9983, 24.6761) centre (30.9983, 24.638) ccw
  line L258 (22.6744, 24.638) -> (21.3257, 24.638)
  arc A516 (21.3257, 24.6761) -> (21.3257, 24.5999) centre (21.3257, 24.638) ccw
  arc A517 (22.6744, 24.5999) -> (22.6744, 24.6761) centre (22.6744, 24.638) ccw
  line L259 (31.0459, 24.7904) -> (29.7064, 24.7904)
  arc A518 (29.7064, 24.8285) -> (29.7064, 24.7523) centre (29.7064, 24.7904) ccw
  arc A519 (31.0459, 24.7523) -> (31.0459, 24.8285) centre (31.0459, 24.7904) ccw
  line L260 (22.6176, 24.7904) -> (21.2782, 24.7904)
  arc A520 (21.2782, 24.8285) -> (21.2782, 24.7523) centre (21.2782, 24.7904) ccw
  arc A521 (22.6176, 24.7523) -> (22.6176, 24.8285) centre (22.6176, 24.7904) ccw
  line L261 (31.0933, 24.9428) -> (29.7633, 24.9428)
  arc A522 (29.7633, 24.9809) -> (29.7633, 24.9047) centre (29.7633, 24.9428) ccw
  arc A523 (31.0933, 24.9047) -> (31.0933, 24.9809) centre (31.0933, 24.9428) ccw
  line L262 (22.5607, 24.9428) -> (21.2307, 24.9428)
  arc A524 (21.2307, 24.9809) -> (21.2307, 24.9047) centre (21.2307, 24.9428) ccw
  arc A525 (22.5607, 24.9047) -> (22.5607, 24.9809) centre (22.5607, 24.9428) ccw
  line L263 (31.1217, 25.0952) -> (29.8191, 25.0952)
  arc A526 (29.8191, 25.1333) -> (29.8191, 25.0571) centre (29.8191, 25.0952) ccw
  arc A527 (31.1217, 25.0571) -> (31.1217, 25.1333) centre (31.1217, 25.0952) ccw
  line L264 (22.5049, 25.0952) -> (21.2023, 25.0952)
  arc A528 (21.2023, 25.1333) -> (21.2023, 25.0571) centre (21.2023, 25.0952) ccw
  arc A529 (22.5049, 25.0571) -> (22.5049, 25.1333) centre (22.5049, 25.0952) ccw
  line L265 (31.1498, 25.2475) -> (29.8523, 25.2476)
  arc A530 (29.8523, 25.2857) -> (29.8523, 25.2095) centre (29.8523, 25.2476) ccw
  arc A531 (31.1498, 25.2094) -> (31.1498, 25.2856) centre (31.1498, 25.2475) ccw
  line L266 (22.4717, 25.2476) -> (21.1744, 25.2476)
  arc A532 (21.1744, 25.2857) -> (21.1744, 25.2095) centre (21.1744, 25.2476) ccw
  arc A533 (22.4717, 25.2095) -> (22.4717, 25.2857) centre (22.4717, 25.2476) ccw
  line L267 (31.1778, 25.3999) -> (29.8854, 25.4)
  arc A534 (29.8854, 25.4381) -> (29.8854, 25.3619) centre (29.8854, 25.4) ccw
  arc A535 (31.1778, 25.3618) -> (31.1778, 25.438) centre (31.1778, 25.3999) ccw
  line L268 (22.4386, 25.4) -> (21.1465, 25.4)
  arc A536 (21.1465, 25.4381) -> (21.1465, 25.3619) centre (21.1465, 25.4) ccw
  arc A537 (22.4386, 25.3619) -> (22.4386, 25.4381) centre (22.4386, 25.4) ccw
  line L269 (31.2051, 25.5524) -> (29.9186, 25.5524)
  arc A538 (29.9186, 25.5905) -> (29.9186, 25.5143) centre (29.9186, 25.5524) ccw
  arc A539 (31.2051, 25.5143) -> (31.2051, 25.5905) centre (31.2051, 25.5524) ccw
  line L270 (22.4054, 25.5524) -> (21.1189, 25.5524)
  arc A540 (21.1189, 25.5905) -> (21.1189, 25.5143) centre (21.1189, 25.5524) ccw
  arc A541 (22.4054, 25.5143) -> (22.4054, 25.5905) centre (22.4054, 25.5524) ccw
  line L271 (31.2139, 25.7047) -> (29.9389, 25.6983)
  arc A542 (29.9389, 25.7364) -> (29.9389, 25.6602) centre (29.9389, 25.6983) ccw
  arc A543 (31.2139, 25.6666) -> (31.2139, 25.7428) centre (31.2139, 25.7047) ccw
  line L272 (22.3847, 25.7048) -> (21.1097, 25.7048)
  arc A544 (21.1097, 25.7429) -> (21.1097, 25.6667) centre (21.1097, 25.7048) ccw
  arc A545 (22.3847, 25.6667) -> (22.3847, 25.7429) centre (22.3847, 25.7048) ccw
  line L273 (31.2224, 25.8572) -> (29.9502, 25.8572)
  arc A546 (29.9502, 25.8953) -> (29.9502, 25.8191) centre (29.9502, 25.8572) ccw
  arc A547 (31.2224, 25.8191) -> (31.2224, 25.8953) centre (31.2224, 25.8572) ccw
  line L274 (22.3738, 25.8572) -> (21.1004, 25.8572)
  arc A548 (21.1004, 25.8953) -> (21.1004, 25.8191) centre (21.1004, 25.8572) ccw
  arc A549 (22.3738, 25.8191) -> (22.3738, 25.8953) centre (22.3738, 25.8572) ccw
  line L275 (31.2308, 26.0096) -> (29.9611, 26.0096)
  arc A550 (29.9611, 26.0477) -> (29.9611, 25.9715) centre (29.9611, 26.0096) ccw
  arc A551 (31.2308, 25.9715) -> (31.2308, 26.0477) centre (31.2308, 26.0096) ccw
  line L276 (22.3629, 26.0096) -> (21.0912, 26.0096)
  arc A552 (21.0912, 26.0477) -> (21.0912, 25.9715) centre (21.0912, 26.0096) ccw
  arc A553 (22.3629, 25.9715) -> (22.3629, 26.0477) centre (22.3629, 26.0096) ccw
  line L277 (31.2392, 26.1619) -> (29.972, 26.162)
  arc A554 (29.972, 26.2001) -> (29.972, 26.1239) centre (29.972, 26.162) ccw
  arc A555 (31.2392, 26.1238) -> (31.2392, 26.2) centre (31.2392, 26.1619) ccw
  line L278 (22.352, 26.162) -> (21.082, 26.162)
  arc A556 (21.082, 26.2001) -> (21.082, 26.1239) centre (21.082, 26.162) ccw
  arc A557 (22.352, 26.1239) -> (22.352, 26.2001) centre (22.352, 26.162) ccw
  line L279 (31.2327, 26.3143) -> (29.9657, 26.3144)
  arc A558 (29.9657, 26.3525) -> (29.9657, 26.2763) centre (29.9657, 26.3144) ccw
  arc A559 (31.2327, 26.2762) -> (31.2327, 26.3524) centre (31.2327, 26.3143) ccw
  line L280 (22.352, 26.3144) -> (21.0956, 26.3144)
  arc A560 (21.0956, 26.3525) -> (21.0956, 26.2763) centre (21.0956, 26.3144) ccw
  arc A561 (22.352, 26.2763) -> (22.352, 26.3525) centre (22.352, 26.3144) ccw
  line L281 (31.2261, 26.4667) -> (29.9593, 26.4668)
  arc A562 (29.9593, 26.5049) -> (29.9593, 26.4287) centre (29.9593, 26.4668) ccw
  arc A563 (31.2261, 26.4286) -> (31.2261, 26.5048) centre (31.2261, 26.4667) ccw
  line L282 (22.3574, 26.4668) -> (21.1092, 26.4668)
  arc A564 (21.1092, 26.5049) -> (21.1092, 26.4287) centre (21.1092, 26.4668) ccw
  arc A565 (22.3574, 26.4287) -> (22.3574, 26.5049) centre (22.3574, 26.4668) ccw
  line L283 (31.2195, 26.6192) -> (29.953, 26.6192)
  arc A566 (29.953, 26.6573) -> (29.953, 26.5811) centre (29.953, 26.6192) ccw
  arc A567 (31.2195, 26.5811) -> (31.2195, 26.6573) centre (31.2195, 26.6192) ccw
  line L284 (22.3736, 26.6192) -> (21.1228, 26.6192)
  arc A568 (21.1228, 26.6573) -> (21.1228, 26.5811) centre (21.1228, 26.6192) ccw
  arc A569 (22.3736, 26.5811) -> (22.3736, 26.6573) centre (22.3736, 26.6192) ccw
  line L285 (31.2129, 26.7716) -> (29.9303, 26.7716)
  arc A570 (29.9303, 26.8097) -> (29.9303, 26.7335) centre (29.9303, 26.7716) ccw
  arc A571 (31.2129, 26.7335) -> (31.2129, 26.8097) centre (31.2129, 26.7716) ccw
  line L286 (22.3898, 26.7716) -> (21.1364, 26.7716)
  arc A572 (21.1364, 26.8097) -> (21.1364, 26.7335) centre (21.1364, 26.7716) ccw
  arc A573 (22.3898, 26.7335) -> (22.3898, 26.8097) centre (22.3898, 26.7716) ccw
  line L287 (31.1912, 26.924) -> (29.9038, 26.924)
  arc A574 (29.9038, 26.9621) -> (29.9038, 26.8859) centre (29.9038, 26.924) ccw
  arc A575 (31.1912, 26.8859) -> (31.1912, 26.9621) centre (31.1912, 26.924) ccw
  line L288 (22.406, 26.924) -> (21.1635, 26.924)
  arc A576 (21.1635, 26.9621) -> (21.1635, 26.8859) centre (21.1635, 26.924) ccw
  arc A577 (22.406, 26.8859) -> (22.406, 26.9621) centre (22.406, 26.924) ccw
  line L289 (31.1637, 27.0764) -> (29.8772, 27.0764)
  arc A578 (29.8772, 27.1145) -> (29.8772, 27.0383) centre (29.8772, 27.0764) ccw
  arc A579 (31.1637, 27.0383) -> (31.1637, 27.1145) centre (31.1637, 27.0764) ccw
  line L290 (22.4425, 27.0764) -> (21.1969, 27.0764)
  arc A580 (21.1969, 27.1145) -> (21.1969, 27.0383) centre (21.1969, 27.0764) ccw
  arc A581 (22.4425, 27.0383) -> (22.4425, 27.1145) centre (22.4425, 27.0764) ccw
  line L291 (31.1361, 27.2288) -> (29.8367, 27.2288)
  arc A582 (29.8367, 27.2669) -> (29.8367, 27.1907) centre (29.8367, 27.2288) ccw
  arc A583 (31.1361, 27.1907) -> (31.1361, 27.2669) centre (31.1361, 27.2288) ccw
  line L292 (22.4812, 27.2288) -> (21.2303, 27.2288)
  arc A584 (21.2303, 27.2669) -> (21.2303, 27.1907) centre (21.2303, 27.2288) ccw
  arc A585 (22.4812, 27.1907) -> (22.4812, 27.2669) centre (22.4812, 27.2288) ccw
  line L293 (31.1086, 27.3812) -> (29.789, 27.3812)
  arc A586 (29.789, 27.4193) -> (29.789, 27.3431) centre (29.789, 27.3812) ccw
  arc A587 (31.1086, 27.3431) -> (31.1086, 27.4193) centre (31.1086, 27.3812) ccw
  line L294 (22.5199, 27.3812) -> (21.2637, 27.3812)
  arc A588 (21.2637, 27.4193) -> (21.2637, 27.3431) centre (21.2637, 27.3812) ccw
  arc A589 (22.5199, 27.3431) -> (22.5199, 27.4193) centre (22.5199, 27.3812) ccw
  line L295 (31.0704, 27.5336) -> (29.7413, 27.5336)
  arc A590 (29.7413, 27.5717) -> (29.7413, 27.4955) centre (29.7413, 27.5336) ccw
  arc A591 (31.0704, 27.4955) -> (31.0704, 27.5717) centre (31.0704, 27.5336) ccw
  line L296 (22.5721, 27.5336) -> (21.3066, 27.5336)
  arc A592 (21.3066, 27.5717) -> (21.3066, 27.4955) centre (21.3066, 27.5336) ccw
  arc A593 (22.5721, 27.4955) -> (22.5721, 27.5717) centre (22.5721, 27.5336) ccw
  line L297 (31.0217, 27.686) -> (29.6795, 27.686)
  arc A594 (29.6795, 27.7241) -> (29.6795, 27.6479) centre (29.6795, 27.686) ccw
  arc A595 (31.0217, 27.6479) -> (31.0217, 27.7241) centre (31.0217, 27.686) ccw
  line L298 (22.635, 27.686) -> (21.3609, 27.686)
  arc A596 (21.3609, 27.7241) -> (21.3609, 27.6479) centre (21.3609, 27.686) ccw
  arc A597 (22.635, 27.6479) -> (22.635, 27.7241) centre (22.635, 27.686) ccw
  line L299 (30.9729, 27.8384) -> (29.6089, 27.8384)
  arc A598 (29.6089, 27.8765) -> (29.6089, 27.8003) centre (29.6089, 27.8384) ccw
  arc A599 (30.9729, 27.8003) -> (30.9729, 27.8765) centre (30.9729, 27.8384) ccw
  line L300 (22.6979, 27.8384) -> (21.4152, 27.8384)
  arc A600 (21.4152, 27.8765) -> (21.4152, 27.8003) centre (21.4152, 27.8384) ccw
  arc A601 (22.6979, 27.8003) -> (22.6979, 27.8765) centre (22.6979, 27.8384) ccw
  line L301 (30.9242, 27.9908) -> (29.5382, 27.9908)
  arc A602 (29.5382, 28.0289) -> (29.5382, 27.9527) centre (29.5382, 27.9908) ccw
  arc A603 (30.9242, 27.9527) -> (30.9242, 28.0289) centre (30.9242, 27.9908) ccw
  line L302 (22.7709, 27.9908) -> (21.4694, 27.9908)
  arc A604 (21.4694, 28.0289) -> (21.4694, 27.9527) centre (21.4694, 27.9908) ccw
  arc A605 (22.7709, 27.9527) -> (22.7709, 28.0289) centre (22.7709, 27.9908) ccw
  line L303 (30.8658, 28.1432) -> (29.449, 28.1432)
  arc A606 (29.449, 28.1813) -> (29.449, 28.1051) centre (29.449, 28.1432) ccw
  arc A607 (30.8658, 28.1051) -> (30.8658, 28.1813) centre (30.8658, 28.1432) ccw
  line L304 (22.8611, 28.1432) -> (21.5324, 28.1432)
  arc A608 (21.5324, 28.1813) -> (21.5324, 28.1051) centre (21.5324, 28.1432) ccw
  arc A609 (22.8611, 28.1051) -> (22.8611, 28.1813) centre (22.8611, 28.1432) ccw
  line L305 (30.7939, 28.2956) -> (29.3523, 28.2956)
  arc A610 (29.3523, 28.3337) -> (29.3523, 28.2575) centre (29.3523, 28.2956) ccw
  arc A611 (30.7939, 28.2575) -> (30.7939, 28.3337) centre (30.7939, 28.2956) ccw
  line L306 (22.9512, 28.2956) -> (21.6096, 28.2956)
  arc A612 (21.6096, 28.3337) -> (21.6096, 28.2575) centre (21.6096, 28.2956) ccw
  arc A613 (22.9512, 28.2575) -> (22.9512, 28.3337) centre (22.9512, 28.2956) ccw
  line L307 (30.7221, 28.448) -> (29.2552, 28.448)
  arc A614 (29.2552, 28.4861) -> (29.2552, 28.4099) centre (29.2552, 28.448) ccw
  arc A615 (30.7221, 28.4099) -> (30.7221, 28.4861) centre (30.7221, 28.448) ccw
  line L308 (23.0543, 28.448) -> (21.6867, 28.448)
  arc A616 (21.6867, 28.4861) -> (21.6867, 28.4099) centre (21.6867, 28.448) ccw
  arc A617 (23.0543, 28.4099) -> (23.0543, 28.4861) centre (23.0543, 28.448) ccw
  line L309 (30.6503, 28.6004) -> (29.1278, 28.6004)
  arc A618 (29.1278, 28.6385) -> (29.1278, 28.5623) centre (29.1278, 28.6004) ccw
  arc A619 (30.6503, 28.5623) -> (30.6503, 28.6385) centre (30.6503, 28.6004) ccw
  line L310 (23.1768, 28.6004) -> (21.7639, 28.6004)
  arc A620 (21.7639, 28.6385) -> (21.7639, 28.5623) centre (21.7639, 28.6004) ccw
  arc A621 (23.1768, 28.5623) -> (23.1768, 28.6385) centre (23.1768, 28.6004) ccw
  line L311 (30.5642, 28.7528) -> (29.0005, 28.7528)
  arc A622 (29.0005, 28.7909) -> (29.0005, 28.7147) centre (29.0005, 28.7528) ccw
  arc A623 (30.5642, 28.7147) -> (30.5642, 28.7909) centre (30.5642, 28.7528) ccw
  line L312 (23.2993, 28.7528) -> (21.8545, 28.7528)
  arc A624 (21.8545, 28.7909) -> (21.8545, 28.7147) centre (21.8545, 28.7528) ccw
  arc A625 (23.2993, 28.7147) -> (23.2993, 28.7909) centre (23.2993, 28.7528) ccw
  line L313 (30.4663, 28.9052) -> (28.8516, 28.9052)
  arc A626 (28.8516, 28.9433) -> (28.8516, 28.8671) centre (28.8516, 28.9052) ccw
  arc A627 (30.4663, 28.8671) -> (30.4663, 28.9433) centre (30.4663, 28.9052) ccw
  line L314 (23.4509, 28.9052) -> (21.9577, 28.9052)
  arc A628 (21.9577, 28.9433) -> (21.9577, 28.8671) centre (21.9577, 28.9052) ccw
  arc A629 (23.4509, 28.8671) -> (23.4509, 28.9433) centre (23.4509, 28.9052) ccw
  line L315 (30.3683, 29.0576) -> (28.6859, 29.0576)
  arc A630 (28.6859, 29.0957) -> (28.6859, 29.0195) centre (28.6859, 29.0576) ccw
  arc A631 (30.3683, 29.0195) -> (30.3683, 29.0957) centre (30.3683, 29.0576) ccw
  line L316 (23.6141, 29.0576) -> (22.061, 29.0576)
  arc A632 (22.061, 29.0957) -> (22.061, 29.0195) centre (22.061, 29.0576) ccw
  arc A633 (23.6141, 29.0195) -> (23.6141, 29.0957) centre (23.6141, 29.0576) ccw
  line L317 (30.2703, 29.21) -> (28.4999, 29.21)
  arc A634 (28.4999, 29.2481) -> (28.4999, 29.1719) centre (28.4999, 29.21) ccw
  arc A635 (30.2703, 29.1719) -> (30.2703, 29.2481) centre (30.2703, 29.21) ccw
  line L318 (23.7973, 29.21) -> (22.1643, 29.21)
  arc A636 (22.1643, 29.2481) -> (22.1643, 29.1719) centre (22.1643, 29.21) ccw
  arc A637 (23.7973, 29.1719) -> (23.7973, 29.2481) centre (23.7973, 29.21) ccw
  line L319 (30.1432, 29.3624) -> (28.2832, 29.3624)
  arc A638 (28.2832, 29.4005) -> (28.2832, 29.3243) centre (28.2832, 29.3624) ccw
  arc A639 (30.1432, 29.3243) -> (30.1432, 29.4005) centre (30.1432, 29.3624) ccw
  line L320 (24.0162, 29.3624) -> (22.2963, 29.3624)
  arc A640 (22.2963, 29.4005) -> (22.2963, 29.3243) centre (22.2963, 29.3624) ccw
  arc A641 (24.0162, 29.3243) -> (24.0162, 29.4005) centre (24.0162, 29.3624) ccw
  line L321 (30.0143, 29.5148) -> (28.0245, 29.5148)
  arc A642 (28.0245, 29.5529) -> (28.0245, 29.4767) centre (28.0245, 29.5148) ccw
  arc A643 (30.0143, 29.4767) -> (30.0143, 29.5529) centre (30.0143, 29.5148) ccw
  line L322 (24.2678, 29.5148) -> (22.4305, 29.5148)
  arc A644 (22.4305, 29.5529) -> (22.4305, 29.4767) centre (22.4305, 29.5148) ccw
  arc A645 (24.2678, 29.4767) -> (24.2678, 29.5529) centre (24.2678, 29.5148) ccw
  line L323 (29.8854, 29.6672) -> (27.7423, 29.6216)
  arc A646 (27.7423, 29.6597) -> (27.7423, 29.5835) centre (27.7423, 29.6216) ccw
  arc A647 (29.8854, 29.6291) -> (29.8854, 29.7053) centre (29.8854, 29.6672) ccw
  line L324 (24.5713, 29.6672) -> (22.5647, 29.6672)
  arc A648 (22.5647, 29.7053) -> (22.5647, 29.6291) centre (22.5647, 29.6672) ccw
  arc A649 (24.5713, 29.6291) -> (24.5713, 29.7053) centre (24.5713, 29.6672) ccw
  line L325 (29.7304, 29.8196) -> (27.563, 29.2165)
  arc A650 (27.563, 29.2546) -> (27.563, 29.1784) centre (27.563, 29.2165) ccw
  arc A651 (29.7304, 29.7815) -> (29.7304, 29.8577) centre (29.7304, 29.8196) ccw
  line L326 (25.0026, 29.8196) -> (22.7253, 29.8196)
  arc A652 (22.7253, 29.8577) -> (22.7253, 29.7815) centre (22.7253, 29.8196) ccw
  arc A653 (25.0026, 29.7815) -> (25.0026, 29.8577) centre (25.0026, 29.8196) ccw
  line L327 (29.5628, 29.972) -> (27.3473, 28.2614)
  arc A654 (27.3093, 28.2639) -> (27.3473, 28.2233) centre (27.3473, 28.2614) ccw
  arc A655 (29.5628, 29.9339) -> (29.5628, 30.0101) centre (29.5628, 29.972) ccw
  line L328 (26.162, 29.972) -> (22.8983, 29.972)
  arc A656 (22.8983, 30.0101) -> (22.8983, 29.9339) centre (22.8983, 29.972) ccw
  arc A657 (26.162, 29.9339) -> (26.162, 30.0101) centre (26.162, 29.972) ccw
  line L329 (29.3951, 30.1244) -> (-0.9498, 30.1244)
  arc A658 (-0.9878, 30.1269) -> (-0.9118, 30.1219) centre (-0.9498, 30.1244) ccw
  arc A659 (29.3951, 30.0863) -> (29.3951, 30.1625) centre (29.3951, 30.1244) ccw
  line L330 (26.162, 30.1244) -> (23.0714, 30.1244)
  arc A660 (23.0714, 30.1625) -> (23.0714, 30.0863) centre (23.0714, 30.1244) ccw
  arc A661 (26.162, 30.0863) -> (26.162, 30.1625) centre (26.162, 30.1244) ccw
  line L331 (27.2302, 31.122) -> (27.0432, 28.2814)
  arc A662 (27.0052, 28.2839) -> (27.0812, 28.2789) centre (27.0432, 28.2814) ccw
  arc A663 (27.2302, 31.0839) -> (27.2302, 31.1601) centre (27.2302, 31.122) ccw
  line L332 (26.162, 30.2768) -> (23.2868, 30.2768)